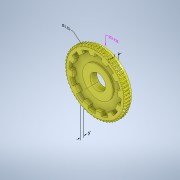
# Autodesk Inventor part: Worm Gear5ForSide
Saved by Autodesk Inventor 2022.2 (Build 262287010, 287A)
## iProperties
CustomPartVersion: 1
Created: 2020-11-06
Part Number: Worm Gear5ForSide
Material: Steel, Mild
Document SubType Name: Modeling
Designer: robst
Categories: <?xml version="1.0" encoding="UTF-16"?> <MemberInstance><Categories><FamilyTemplate><FamilyTemplateParameter ValueType="xs:double" Id="1" ObjectReferenceKey="da_z" ObjectType="kUserParameterObject"/><FamilyTemplateParameter ValueType="xs:double" Id="2" ObjectReferenceKey="da_b" ObjectType="kUserParameterObject"/><FamilyTemplateParameter ValueType="xs:double" Id="3" ObjectReferenceKey="da_beta" ObjectType="kUserParameterObject"/><FamilyTemplateParameter ValueType="xs:double" Id="4" ObjectReferenceKey="da_m" ObjectType="kUserParameterObject"/><FamilyTemplateParameter ValueType="xs:double" Id="5" ObjectReferenceKey="da_alpha" ObjectType="kUserParameterObject"/><FamilyTemplateParameter ValueType="xs:double" Id="6" ObjectReferenceKey="da_da" ObjectType="kUserParameterObject"/><FamilyTemplateParameter ValueType="xs:double" Id="7" ObjectReferenceKey="da_aw" ObjectType="kUserParameterObject"/><FamilyTemplateParameter ValueType="xs:double" Id="8" ObjectReferenceKey="da_px" ObjectType="kUserParameterObject"/><FamilyTemplateParameter ValueType="xs:double" Id="9" ObjectReferenceKey="da_d" ObjectType="kUserParameterObject"/><FamilyTemplateParameter ValueType="xs:double" Id="10" ObjectReferenceKey="da_dae" ObjectType="kUserParameterObject"/><FamilyTemplateParameter ValueType="xs:double" Id="11" ObjectReferenceKey="da_fi" ObjectType="kUserParameterObject"/><FamilyTemplateParameter ValueType="xs:string" Id="12" ObjectReferenceKey="EAIAABAAAAAWFwAAAAAAAIAAAAAAAAAA" ObjectType="83910656" SubObjectId="SurfaceGeometry"/></FamilyTemplate><ParamToTemplateMap><ParamToTemplate CategoryParameter="//CategoryParameter[@InternalName='046C89C9-8512-4d59-83FE-43B91F4F132A']" TemplateParameter="1"/><ParamToTemplate CategoryParameter="//CategoryParameter[@InternalName='2552DF32-E462-4b46-AEBF-C6C7768E72AC']" TemplateParameter="2"/><ParamToTemplate CategoryParameter="//CategoryParameter[@InternalName='C9EE641D-15FC-4fae-A226-E94C4372FDD7']" TemplateParameter="3"/><ParamToTemplate><ParamToTemplate CategoryParameter="//CategoryParameter[@InternalName='00B6519A-459B-49c7-AD84-2E56D39A5744']" ConstantValue="0.000000"/></ParamToTemplate><ParamToTemplate><ParamToTemplate CategoryParameter="//CategoryParameter[@InternalName='04B31F0E-C7A6-4894-AA32-9629BEFACF47']" ConstantValue="1.000000"/></ParamToTemplate><ParamToTemplate><ParamToTemplate CategoryParameter="//CategoryParameter[@InternalName='43CBEC2E-7847-49e7-A936-2F7889FCB2D9']" ConstantValue="0.200000"/></ParamToTemplate><ParamToTemplate><ParamToTemplate CategoryParameter="//CategoryParameter[@InternalName='B1EFC894-105D-4ebd-86BF-FA20ED196853']" ConstantValue="0.300000"/></ParamToTemplate><ParamToTemplate><ParamToTemplate CategoryParameter="//CategoryParameter[@InternalName='51175063-3D10-4879-93E8-6246FE8B403D']" ConstantValue="2061532430.657340"/></ParamToTemplate><ParamToTemplate><ParamToTemplate CategoryParameter="//CategoryParameter[@InternalName='A3A52E27-4454-46a9-B0BD-C932399B70AF']" ConstantValue="0.300000"/></ParamToTemplate><ParamToTemplate CategoryParameter="//CategoryParameter[@InternalName='91B76062-C214-41d9-B1B9-14D2AB99603D']" TemplateParameter="4"/><ParamToTemplate CategoryParameter="//CategoryParameter[@InternalName='2D373A89-B862-43d6-8D0B-0CBF12AB9F6C']" TemplateParameter="5"/><ParamToTemplate CategoryParameter="//CategoryParameter[@InternalName='37777632-D6A2-4fac-9D53-DB8ACD95C989']" TemplateParameter="6"/><ParamToTemplate CategoryParameter="//CategoryParameter[@InternalName='FD1017F1-B727-4f7e-9707-0F86F1FF9423']" TemplateParameter="7"/><ParamToTemplate CategoryParameter="//CategoryParameter[@InternalName='3BF567DA-17EF-48d8-80EA-D119B07F6463']" TemplateParameter="8"/><ParamToTemplate CategoryParameter="//CategoryParameter[@InternalName='BF5A1E7E-5373-4a22-AAD3-F583781FCF3C']" TemplateParameter="9"/><ParamToTemplate CategoryParameter="//CategoryParameter[@InternalName='2A200944-5A8C-41ca-B96E-8520D2E510F1']" TemplateParameter="10"/><ParamToTemplate CategoryParameter="//CategoryParameter[@InternalName='E77AC4FD-7B43-4566-B0ED-7CA70B976BC8']" TemplateParameter="11"/><ParamToTemplate><ParamToTemplate CategoryParameter="//CategoryParameter[@InternalName='D4F72237-D604-435a-AD0B-F738B7463A00']" ConstantValue="110.000000"/></ParamToTemplate><ParamToTemplate><ParamToTemplate CategoryParameter="//CategoryParameter[@InternalName='9E1B4470-B2D3-4ff1-B813-535BB4CDF51A']" ConstantValue="1999479.615019"/></ParamToTemplate><ParamToTemplate><ParamToTemplate CategoryParameter="//CategoryParameter[@InternalName='A7A89E9A-52E6-4d4f-86CF-A81914F22AA4']" ConstantValue="250000000.000000"/></ParamToTemplate><ParamToTemplate><ParamToTemplate CategoryParameter="//CategoryParameter[@InternalName='B02FABAC-469F-4ad8-A219-DB4578299DF6']" ConstantValue="250000000.000000"/></ParamToTemplate><ParamToTemplate><ParamToTemplate CategoryParameter="//CategoryParameter[@InternalName='E6981962-40D5-4343-A0AD-C263FCC47E10']" ConstantValue="9.000000"/></ParamToTemplate><ParamToTemplate><ParamToTemplate CategoryParameter="//CategoryParameter[@InternalName='B958E99F-2BCD-4955-8634-793EB7B37B89']" ConstantValue="8.000000"/></ParamToTemplate><ParamToTemplate><ParamToTemplate CategoryParameter="//CategoryParameter[@InternalName='4AD49A87-569D-440f-A541-E3B52A6A9DCE']" ConstantValue="1219.200000"/></ParamToTemplate><ParamToTemplate><ParamToTemplate CategoryParameter="//CategoryParameter[@InternalName='4E5813A0-330D-4b41-BE23-D880B01A1D55']" ConstantValue="1654741.750360"/></ParamToTemplate><ParamToTemplate><ParamToTemplate CategoryParameter="//CategoryParameter[@InternalName='19EB8C86-AA88-4253-B4AA-2F5DF1CE171A']" ConstantValue="5515.805835"/></ParamToTemplate><ParamToTemplate CategoryParameter="//CategoryParameter[@InternalName='27C3BAF2-7550-4e4b-AE2C-0DB134B7D9B7']" TemplateParameter="12"/></ParamToTemplateMap><Category DisplayName="Gear" InternalName="DC85795E-93AB-48d5-8EEE-5A27447B64BD" Mnemonic="Gear"><CategoryParameter DisplayName="z" InternalName="046C89C9-8512-4d59-83FE-43B91F4F132A" Mnemonic="z"/><CategoryParameter DisplayName="b|.2|" InternalName="2552DF32-E462-4b46-AEBF-C6C7768E72AC" Mnemonic="b"/><CategoryParameter DisplayName="||b|" InternalName="C9EE641D-15FC-4fae-A226-E94C4372FDD7" Mnemonic="beta"/><CategoryParameter DisplayName="x" InternalName="00B6519A-459B-49c7-AD84-2E56D39A5744" Mnemonic="x"/><CategoryParameter DisplayName="a*" InternalName="04B31F0E-C7A6-4894-AA32-9629BEFACF47" Mnemonic="a"/><CategoryParameter DisplayName="c*" InternalName="43CBEC2E-7847-49e7-A936-2F7889FCB2D9" Mnemonic="c"/><CategoryParameter DisplayName="r|.f|*" InternalName="B1EFC894-105D-4ebd-86BF-FA20ED196853" Mnemonic="rf"/><CategoryParameter DisplayName="E" InternalName="51175063-3D10-4879-93E8-6246FE8B403D" Mnemonic="E"/><CategoryParameter DisplayName="||m|" InternalName="A3A52E27-4454-46a9-B0BD-C932399B70AF" Mnemonic="mi"/><Category DisplayName="WormGear" InternalName="1B25C7EF-093B-4025-B3D3-619CD2A4550C" Mnemonic="WormGear"><CategoryParameter DisplayName="m" InternalName="91B76062-C214-41d9-B1B9-14D2AB99603D" Mnemonic="m"/><CategoryParameter DisplayName="||a|" InternalName="2D373A89-B862-43d6-8D0B-0CBF12AB9F6C" Mnemonic="alpha"/><CategoryParameter DisplayName="d|.a|" InternalName="37777632-D6A2-4fac-9D53-DB8ACD95C989" Mnemonic="da"/><CategoryParameter DisplayName="a|.w|" InternalName="FD1017F1-B727-4f7e-9707-0F86F1FF9423" Mnemonic="aw"/><CategoryParameter DisplayName="p|.x|" InternalName="3BF567DA-17EF-48d8-80EA-D119B07F6463" Mnemonic="px"/><CategoryParameter DisplayName="d" InternalName="BF5A1E7E-5373-4a22-AAD3-F583781FCF3C" Mnemonic="d"/><CategoryParameter DisplayName="dae" InternalName="2A200944-5A8C-41ca-B96E-8520D2E510F1" Mnemonic="dae"/><CategoryParameter DisplayName="||d|" InternalName="E77AC4FD-7B43-4566-B0ED-7CA70B976BC8" Mnemonic="fi"/><CategoryParameter DisplayName="VHV" InternalName="D4F72237-D604-435a-AD0B-F738B7463A00" Mnemonic="VHV"/><CategoryParameter DisplayName="||s||.Hlim|" InternalName="9E1B4470-B2D3-4ff1-B813-535BB4CDF51A" Mnemonic="sHlim"/><CategoryParameter DisplayName="N|.Flim|" InternalName="A7A89E9A-52E6-4d4f-86CF-A81914F22AA4" Mnemonic="NFlim"/><CategoryParameter DisplayName="N|.Hlim|" InternalName="B02FABAC-469F-4ad8-A219-DB4578299DF6" Mnemonic="NHlim"/><CategoryParameter DisplayName="q|.F|" InternalName="E6981962-40D5-4343-A0AD-C263FCC47E10" Mnemonic="qF"/><CategoryParameter DisplayName="q|.H|" InternalName="B958E99F-2BCD-4955-8634-793EB7B37B89" Mnemonic="qH"/><CategoryParameter DisplayName="v|.max|" InternalName="4AD49A87-569D-440f-A541-E3B52A6A9DCE" Mnemonic="maxv"/><CategoryParameter DisplayName="S|.n|" InternalName="4E5813A0-330D-4b41-BE23-D880B01A1D55" Mnemonic="Sn"/><CategoryParameter DisplayName="K|.w|" InternalName="19EB8C86-AA88-4253-B4AA-2F5DF1CE171A" Mnemonic="Kw"/><CategoryParameter DisplayName="PitchDiameter" InternalName="27C3BAF2-7550-4e4b-AE2C-0DB134B7D9B7" Mnemonic="IDS_PITCHDIAM"/></Category></Category></Categories></MemberInstance>
Density: 7.86 g/cm^3
Appearance: Yellow
Author: robst
Autodesk Inventor part; units mm, degrees
ref_plane "Tooth Plane" through (0, -10, 0) normal (-0.0995037, 0, 0.9950372) x (0, 1, 0)
sketch "Base Body Sketch" plane through (0, 0, 0) normal (1, 0, 0) x (0, 1, 0)
  line L0 (0, -9.0553) -> (0, 9.0553) projected
  line L1 (0, 4.7625) -> (48.1427, 4.7625)
  line L2 (48.1427, 4.7625) -> (50.9359, 3.1887)
  line L3 (-58.447, 0) -> (83.3153, 0) construction
  circle A0 centre (56.5955, 0) radius 6.4681
  line L4 (50.9359, 3.1887) -> (50.9359, -3.1887)
  line L5 (0, -4.7625) -> (48.1427, -4.7625)
  line L6 (0, 4.7625) -> (0, -4.7625)
  line L7 (48.1427, -4.7625) -> (50.9359, -3.1887)
  dimension "d50" = 29.398
  dimension "d87" = 101.8719
  dimension "d89" = 12.9361
  dimension "d92" = 9.525
  dimension "d93" = 56.5955
  constraints: 14 end point, 3 symmetric about line, 2 perpendicular, 2 point on line, 1 centre point, 1 collinear
  measures "d50" angle of L2 L1
  measures "d87" diameter of L4 L0
  measures "d89" diameter of A0
  measures "d92" distance of L1.start L5.start
  measures "d93" distance from line of A0.centre L6
revolve "Base Body" add sketch "Base Body Sketch" angle 360 about axis through (0, 0, 0) along (0, 0, 1) picked at (50.7648, 0.6438) contours L0 L1 L2 L4 A0 L7 L5 | A0 L4
revolve "Base Body2" cut sketch "Base Body Sketch" angle 360 about axis through (0, 0, 0) along (0, 0, 1) contours L4 A0 | A0 L4
sketch "Tooth Sketch" plane through (0, -10, 0) normal (-0.0995037, 0, 0.9950372) x (0, 1, 0)
  line L0 (10, 53.3292) -> (10, -53.7811) projected
  line L1 (-66.6726, 0) -> (73.8669, 0) projected
  line L2 (-46.5955, 2.2303) -> (-46.5955, -2.2303)
  line L3 (-46.5955, -2.2303) -> (-40.4508, -2.2303)
  line L4 (-40.4508, -2.2303) -> (-36.57, -0.8177)
  line L5 (-36.57, -0.8177) -> (-36.57, 0)
  line L6 (-36.57, 0.8177) -> (-40.4508, 2.2303)
  line L7 (-40.4508, 2.2303) -> (-46.5955, 2.2303)
  line L8 (-36.57, 0.8177) -> (-36.57, 0)
  line L9 (-38.5104, 0) -> (-38.5104, -1.524) construction
  dimension "d38" = 56.5955
  dimension "d39" = 20
  dimension "d40" = 6.1447
  dimension "d41" = 8.0851
  dimension "d42" = 1.524
  constraints: 16 end point, 4 perpendicular, 3 equal length, 2 point on line, 1 midpoint, 1 parallel, 1 vertical
  measures "d38" distance between parallel lines of L0 L2
  measures "d39" angle of L6 L7
  measures "d40" distance of L6.end L2.start
  measures "d41" distance between parallel lines of L2 L9
  measures "d42" distance of L9.start L9.end
sketch "Sketch8" plane through (0, 0, 4.7625) normal (0, 0, 1) x (1, 0, 0)
  circle A0 centre (0, 0) radius 48.1427 projected
  circle A1 centre (0, 0) radius 48.5104
  dimension "d77" = 97.0208
  constraints: 1 centre point, 1 coincident
  measures "d77" diameter of A1
surface extrude "Pitch Diameter" sketch "Sketch8" against normal blind 9.525 shown no curves A1
ref_plane "Work Plane13" through (0, 0, 0) normal (-0.052336, 0.9986295, 0) x (0, 0, 1)
revolve "Tooth" cut sketch "Tooth Sketch" angle 360 about axis through (-2.2192, -56.5955, -0.2219) along (0.9950372, 0, 0.0995037)
pattern_circular "Tooth Pattern" count 60 over 360 about axis through (0, 0, 0) along (0, 0, 1) of "Tooth"
ref_plane "Work Plane14" through (0, 0, 0) normal (0.9986295, 0.052336, 0) x (0, 0, 1)
ref_plane "Work Plane15" through (0, 0, 0) normal (0, -1, 0) x (0, 0, 1)
sketch "Sketch10" plane through (47.625, -56.5955, 4.7625) normal (0, 0, 1) x (1, 0, 0)
  circle A0 centre (-47.625, 56.5955) radius 38.1953
  dimension "d97" = 76.3905
  constraints: 1 centre point, 1 coincident
  measures "d97" diameter of A0
extrude "Extrusion2" cut sketch "Sketch10" against normal through all
sketch "Sketch11" plane through (-47.625, -56.5955, -4.7625) normal (0, 0, -1) x (-1, 0, 0)
  circle A0 centre (-47.625, 56.5955) radius 12.8905
  circle A1 centre (-47.625, 56.5955) radius 47.4345
  dimension "d102" = 25.781
  dimension "d103" = 94.869
  constraints: 2 centre point, 2 coincident
  measures "d102" diameter of A0
  measures "d103" diameter of A1
extrude "Extrusion3" add sketch "Sketch11" along normal blind 6.35
sketch "Sketch16" plane through (47.625, -56.5955, 4.7625) normal (0, 0, 1) x (1, 0, 0)
  circle A0 centre (-47.625, 56.5955) radius 38.1953 projected
  arc A1 (-37.4178, 93.4016) -> (-47.9583, 94.7893) centre (-47.625, 56.5955) ccw
  arc A2 (-36.0341, 98.3911) -> (-48.0035, 99.9669) centre (-47.625, 56.5955) ccw
  circle A3 centre (-47.625, 56.5955) radius 12.8905 construction
  line L0 (-47.625, 56.5955) -> (-47.625, 99.9685) construction
  line L1 (-47.9583, 94.7893) -> (-48.0035, 99.9669)
  line L2 (-37.4178, 93.4016) -> (-36.0341, 98.3911)
  point P0 (-47.9583, 94.7893)
  dimension "d159" = 76.3905
  dimension "d153" = 5.1778
  dimension "d160" = 86.7461
  constraints: 6 end point, 5 point on circle, 2 centre point, 2 coincident, 1 vertical, 3 other
  measures "d160" diameter of A2
extrude "Extrusion7" cut sketch "Sketch16" against normal blind 9.525 contours A0 L1 A2 L2
pattern_circular "Circular Pattern7" count 12 over 360 about axis through (0, 0, 0) along (0, 0, 1) of "Extrusion7"
sketch "Sketch17" plane through (-47.625, -56.5955, -4.7625) normal (0, 0, 1) x (1, 0, 0)
  circle A0 centre (47.625, 56.5955) radius 12.8905 projected
  circle A1 centre (47.625, 56.5955) radius 12.8905 projected
  circle A2 centre (47.625, 56.5955) radius 12.8905
  circle A3 centre (47.625, 56.5955) radius 25.4
  dimension "d168" = 50.8
  constraints: 2 centre point, 2 coincident
  measures "d168" diameter of A3
extrude "Extrusion8" add sketch "Sketch17" along normal blind 4.7625
sketch "Sketch18" plane through (0, 0, -11.1125) normal (0, 0, -1) x (-1, 0, 0)
  circle A0 centre (0, 0) radius 44.45 construction
  circle A1 centre (0, 0) radius 49.53
  circle A2 centre (0, 0) radius 39.37
  dimension "d171" = 88.9
  dimension "d172" = 5.08
  dimension "d173" = 5.08
  constraints: 3 centre point, 3 coincident
  measures "d171" diameter of A0
  measures "d172" radial gap between concentric circles of A1 A0
  measures "d173" radial gap between concentric circles of A0 A2
extrude "Extrusion9" cut sketch "Sketch18" against normal blind 2.54
sketch "Sketch19" plane through (-47.625, -56.5955, -4.7625) normal (0, 0, 1) x (1, 0, 0)
  circle A0 centre (47.625, 56.5955) radius 25.4 projected
  circle A1 centre (47.625, 56.5955) radius 25.4
  circle A2 centre (47.625, 56.5955) radius 43.3793
  constraints: 2 centre point, 2 coincident, 1 concentric
extrude "Extrusion10" add sketch "Sketch19" along normal blind 3.175
equation "\"d50\" = da_fi"
equation "\"d87\" = da_dae"
equation "\"d89\" = 2 * da_aw - da_da"
equation "\"d92\" = da_b"
equation "\"d93\" = da_aw"
equation "\"d97\" = interiorHoleDiameter + printSpacing"
equation "\"d102\" = shaftHoleDiameter + 2 * printSpacing"
equation "\"d153\" = depthForSpline"
equation "\"d38\" = da_aw"
equation "\"d39\" = da_alfat"
equation "\"d40\" = 0.5 * da_df1"
equation "\"d41\" = 0.5 * da_d1"
equation "\"d42\" = 0.3 * da_px"
equation "\"d77\" = da_dw"
equation "\"d78\" = da_b"
equation "\"da_aw\" = 56.5955"
equation "\"da_fi\" = 29.398deg"
equation "\"da_b\" = 9.525"
equation "\"da_df\" = 93.14002"
equation "\"da_da\" = 100.25488"
equation "\"da_beta\" = 5.710593deg"
equation "\"da_alfat\" = 20deg"
equation "\"da_df1\" = 12.28931"
equation "\"da_da1\" = 19.40417"
equation "\"da_d1\" = 16.17014"
equation "\"da_px\" = 5.08"
equation "\"d68\" = da_aw"
equation "\"da_dw\" = 97.02085"
equation "\"da_rightdir\" = 0"
equation "\"d86\" = da_aw"
equation "\"da_dae\" = 101.8719"
equation "\"interiorHoleDiameter\" = 76.2"
equation "\"pi\" = 3.141593"
equation "\"diameterForSplines\" = 76.2"
equation "\"depthForSpline\" = 0.5 * widthOfSpline + printSpacing"
equation "\"shaftHoleDiameter\" = 25.4"
equation "\"printSpacing\" = 0.1905"
equation "\"printSpacingAngleDiff\" = 1deg"
equation "\"absPrintSpacingAngleDiff\" = printSpacingAngleDiff"
equation "\"d151\" = 0.5 * absPrintSpacingAngleDiff"
equation "\"d152\" = angleForSplineTooth"
equation "\"widthOfSpline\" = 9.974557"
equation "\"angleForSplineTooth\" = 16deg"
body "Solid1"
body "Srf1"
